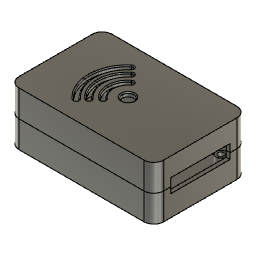
diymore (Autodesk Fusion 360 design; units mm, degrees)
Autodesk Fusion 360 part; units mm, degrees
note: some values were not read from the file. Chosen so that the rebuilt part matches the saved one: which face or edge a step refers to. Set by a fixed rule: which sketch regions a step uses.
sketch "Sketch1" plane through (0, 0, 0) normal (0, 0, 1) x (1, 0, 0) in component "Case"
  line L0 (36.5556, -23.5) -> (-36.5556, -23.5)
  line L1 (-36.5556, -23.5) -> (-36.5556, 23.5)
  line L2 (-36.5556, 23.5) -> (36.5556, 23.5)
  line L3 (36.5556, 23.5) -> (36.5556, -23.5)
  line L4 (36.5556, -23.5) -> (-36.5556, 23.5) construction
  line L5 (-36.5556, -23.5) -> (36.5556, 23.5) construction
  dimension "d4" = 47
  constraint horizontal L0
  constraint perpendicular L0 L1
  constraint parallel L0 L2
  constraint parallel L1 L3
  constraint coincident L4 origin
  constraint coincident L5 origin
  measures "d4" distance of L0.end L1.end
extrude "Extrude1" add sketch "Sketch1" along normal blind 27 makes body 1 in component "Case"
fillet "Fillet1" radius 5 4 edges at (36.5556, -23.5, 13.5) (36.5556, 23.5, 13.5) (-36.5556, -23.5, 13.5) (-36.5556, 23.5, 13.5) on bodies 1 in component "Case"
shell "Shell1" thickness 2 removed faces 0 bodies 1 in component "Case"
ref_plane "WorkPlane1" through (0, 0, 13.5) normal (0, 0, 1) x (1, 0, 0) in component "Case"
sketch "Sketch3" plane through (36.5556, 0, 0) normal (1, 0, 0) x (0, 1, 0) in component "Case"
  line L0 (-18.5, 27) -> (-18.5, 0)
  line L1 (18.5, 0) -> (18.5, 27)
  line L2 (0, 0) -> (0, 7) construction
  line L3 (0, 7) -> (15, 7) construction
  line L4 (0, 7) -> (0, 13.5) construction
  line L5 (0, 7) -> (-15, 7) construction
  line L6 (-13.9847, 14) -> (14, 14) construction
  line L7 (15.0076, 10.5) -> (-14.9924, 10.5)
  line L8 (-14.9924, 10.5) -> (-14.9924, 17.5)
  line L9 (-14.9924, 17.5) -> (15.0076, 17.5)
  line L10 (15.0076, 17.5) -> (15.0076, 10.5)
  line L11 (15.0076, 10.5) -> (-14.9924, 17.5) construction
  line L12 (-14.9924, 10.5) -> (15.0076, 17.5) construction
  line L13 (18.5, 27) -> (-18.5, 27)
  line L14 (-18.5, 0) -> (18.5, 0)
  point P0 (0.0076, 14)
  dimension "d19" = 7
  dimension "d20" = 15
  dimension "d21" = 15
  dimension "d24" = 30
  dimension "d25" = 7
  constraint coincident L2.start origin
  constraint perpendicular L2 L3
  constraint perpendicular L2 L5
  constraint horizontal L6
  constraint horizontal L7
  constraint perpendicular L7 L8
  constraint parallel L7 L9
  constraint parallel L8 L10
  constraint coincident L11 P0
  constraint coincident L12 P0
  constraint midpoint L6 P0
  measures "d19" distance of L2.start L2.end
  measures "d20" distance of L2.end L3.end
  measures "d21" distance of L2.end L5.end
  measures "d24" distance of L8.end L9.end
  measures "d25" distance of L7.end L8.end
extrude "Extrude10" cut sketch "Sketch3" against normal blind 15 contours L7 L8 L9 L10 bodies 1 in component "Case"
sketch "Sketch10" plane through (-36.5556, 0, 0) normal (-1, 0, 0) x (0, -1, 0) in component "Case"
  line L0 (18.5, 0) -> (18.5, 27)
  line L1 (-18.5, 27) -> (-18.5, 0)
  line L2 (14.9924, 17.5) -> (-15.0076, 17.5)
  line L3 (-15.0076, 10.5) -> (14.9924, 10.5)
  line L4 (-5, 17.5) -> (5, 17.5)
  line L5 (5, 17.5) -> (5, 10.5)
  line L6 (5, 10.5) -> (-5, 10.5)
  line L7 (-5, 10.5) -> (-5, 17.5)
  line L8 (-5, 17.5) -> (5, 10.5) construction
  line L9 (5, 17.5) -> (-5, 10.5) construction
  line L10 (-18.5, 0) -> (18.5, 0)
  line L11 (18.5, 27) -> (-18.5, 27)
  point P0 (0, 14)
  dimension "d75" = 10
  constraint horizontal L4
  constraint perpendicular L4 L5
  constraint parallel L4 L6
  constraint parallel L5 L7
  constraint coincident L8 P0
  constraint coincident L9 P0
  measures "d75" distance of L5.end L6.end
extrude "Extrude11" cut sketch "Sketch10" against normal blind 15 contours L2 L3 L4 L5 L6 L7 bodies 1 in component "Case"
split "Split1" by plane through (0, 0, 13.5) normal (0, 0, 1) bodies 1 makes body 2 at (-10.5185, -7.8333, 27) in component "Case"
sketch "Sketch2" plane through (0, 0, 2) normal (0, 0, 1) x (-1, 0, 0) in component "Case"
  circle A0 centre (30, 18) radius 1.5
  circle A1 centre (30, 18) radius 2.5
  circle A2 centre (-29.4798, -17.5013) radius 1.5
  circle A3 centre (-29.4798, -17.5013) radius 2.5
  circle A4 centre (30, -18) radius 1.5
  line L0 (-29.4798, -17.5013) -> (-29.4798, 19.4069) construction
  circle A5 centre (-29.4798, 17.9693) radius 1.5
  arc A6 (-31.5556, 21.5) -> (-34.5556, 18.5) centre (-31.5556, 18.5) ccw
  line L1 (-34.5556, 18.5) -> (-34.5556, -18.5)
  arc A7 (-34.5556, -18.5) -> (-31.5556, -21.5) centre (-31.5556, -18.5) ccw
  line L2 (-31.5556, -21.5) -> (31.5556, -21.5)
  arc A8 (31.5556, -21.5) -> (34.5556, -18.5) centre (31.5556, -18.5) ccw
  line L3 (34.5556, -18.5) -> (34.5556, 18.5)
  arc A9 (34.5556, 18.5) -> (31.5556, 21.5) centre (31.5556, 18.5) ccw
  line L4 (31.5556, 21.5) -> (-31.5556, 21.5)
  dimension "d10" = 3
  dimension "d11" = 1
  dimension "d12" = 3
  dimension "d13" = 1
  dimension "d14" = 3
  dimension "d16" = 3
  constraint coincident A2.centre A3.centre
  constraint vertical L0
  constraint coincident L0 A5.centre
  measures "d10" diameter of A0
  measures "d12" diameter of A2
  measures "d14" diameter of A4
  measures "d16" diameter of A5
extrude "Extrude2" add sketch "Sketch2" along normal blind 6 contours A1 | A3 | A4 | A5 bodies 1 in component "Case"
sketch "Sketch5" plane through (0, 23.5, 0) normal (0, 1, 0) x (-1, 0, 0) in component "Case"
  line L0 (-31.5556, 13.5) -> (-31.5556, 0)
  line L1 (31.5556, 0) -> (31.5556, 13.5)
  line L2 (20.224, 13.5) -> (20.224, 9.5) construction
  line L3 (20.224, 9.5) -> (26.224, 9.5)
  line L4 (26.224, 9.5) -> (26.224, 6.5)
  line L5 (26.224, 6.5) -> (20.224, 6.5)
  line L6 (20.224, 6.5) -> (20.224, 9.5)
  line L7 (31.5556, 13.5) -> (-31.5556, 13.5)
  line L8 (-31.5556, 0) -> (31.5556, 0)
  dimension "d32" = 4
  dimension "d33" = 6
  dimension "d34" = 3
  constraint horizontal L3
  constraint vertical L4
  constraint horizontal L5
  constraint vertical L6
  measures "d32" distance of L2.start L2.end
  measures "d33" distance of L2.end L3.end
  measures "d34" distance of L2.end L5.end
sketch "Sketch7" plane through (0, 0, 13.5) normal (0, 0, 1) x (-1, 0, 0) in component "Case"
  arc A0 (35.0556, 18.5) -> (31.5556, 22) centre (31.5556, 18.5) ccw
  line L0 (-31.5556, 22) -> (31.5556, 22)
  arc A1 (-31.5556, 22) -> (-35.0556, 18.5) centre (-31.5556, 18.5) ccw
  line L1 (-35.0556, 15.4924) -> (-35.0556, 18.5)
  line L2 (-36.0556, 15.4924) -> (-35.0556, 15.4924)
  line L3 (-36.0556, 18.5) -> (-36.0556, 15.4924)
  arc A2 (-31.5556, 23) -> (-36.0556, 18.5) centre (-31.5556, 18.5) ccw
  line L4 (31.5556, 23) -> (-31.5556, 23)
  arc A3 (36.0556, 18.5) -> (31.5556, 23) centre (31.5556, 18.5) ccw
  line L5 (36.0556, 5.5) -> (36.0556, 18.5)
  line L6 (35.0556, 5.5) -> (36.0556, 5.5)
  line L7 (35.0556, 18.5) -> (35.0556, 5.5)
  arc A4 (36.5556, 18.5) -> (31.5556, 23.5) centre (31.5556, 18.5) ccw
  line L8 (31.5556, 23.5) -> (-31.5556, 23.5)
  arc A5 (-31.5556, 23.5) -> (-36.5556, 18.5) centre (-31.5556, 18.5) ccw
  line L9 (-36.5556, 18.5) -> (-36.5556, 14.9924)
  line L10 (-36.5556, 14.9924) -> (-34.5556, 14.9924)
  line L11 (-34.5556, 14.9924) -> (-34.5556, 18.5)
  arc A6 (-31.5556, 21.5) -> (-34.5556, 18.5) centre (-31.5556, 18.5) ccw
  line L12 (-31.5556, 21.5) -> (31.5556, 21.5)
  arc A7 (34.5556, 18.5) -> (31.5556, 21.5) centre (31.5556, 18.5) ccw
  line L13 (34.5556, 18.5) -> (34.5556, 5)
  line L14 (34.5556, 5) -> (36.5556, 5)
  line L15 (36.5556, 5) -> (36.5556, 18.5)
  constraint tangent A0 L0
  constraint tangent A1 L1
  constraint tangent L4 A3
  constraint tangent A3 L5
  constraint tangent L3 A2
  constraint tangent L0 A1
  constraint tangent A2 L4
  constraint tangent A0 L7
sketch "Sketch8" plane through (0, 0, 13.5) normal (0, 0, 1) x (-1, 0, 0) in component "Case"
  arc A0 (-35.0556, -18.5) -> (-31.5556, -22) centre (-31.5556, -18.5) ccw
  line L0 (31.5556, -22) -> (-31.5556, -22)
  arc A1 (31.5556, -22) -> (35.0556, -18.5) centre (31.5556, -18.5) ccw
  line L1 (35.0556, -5.5) -> (35.0556, -18.5)
  line L2 (36.0556, -5.5) -> (35.0556, -5.5)
  line L3 (36.0556, -18.5) -> (36.0556, -5.5)
  arc A2 (31.5556, -23) -> (36.0556, -18.5) centre (31.5556, -18.5) ccw
  line L4 (-31.5556, -23) -> (31.5556, -23)
  arc A3 (-36.0556, -18.5) -> (-31.5556, -23) centre (-31.5556, -18.5) ccw
  line L5 (-36.0556, -15.5076) -> (-36.0556, -18.5)
  line L6 (-35.0556, -15.5076) -> (-36.0556, -15.5076)
  line L7 (-35.0556, -18.5) -> (-35.0556, -15.5076)
  arc A4 (31.5556, -23.5) -> (36.5556, -18.5) centre (31.5556, -18.5) ccw
  line L8 (36.5556, -18.5) -> (36.5556, -5)
  line L9 (36.5556, -5) -> (34.5556, -5)
  line L10 (34.5556, -5) -> (34.5556, -18.5)
  arc A5 (31.5556, -21.5) -> (34.5556, -18.5) centre (31.5556, -18.5) ccw
  line L11 (31.5556, -21.5) -> (-31.5556, -21.5)
  arc A6 (-34.5556, -18.5) -> (-31.5556, -21.5) centre (-31.5556, -18.5) ccw
  line L12 (-34.5556, -18.5) -> (-34.5556, -15.0076)
  line L13 (-34.5556, -15.0076) -> (-36.5556, -15.0076)
  line L14 (-36.5556, -15.0076) -> (-36.5556, -18.5)
  arc A7 (-36.5556, -18.5) -> (-31.5556, -23.5) centre (-31.5556, -18.5) ccw
  line L15 (-31.5556, -23.5) -> (31.5556, -23.5)
  constraint tangent L3 A2
  constraint tangent A3 L5
  constraint tangent A1 L1
  constraint tangent A0 L0
  constraint tangent A0 L7
  constraint tangent L0 A1
  constraint tangent A2 L4
  constraint tangent L4 A3
extrude "Extrude7" add sketch "Sketch8" sketch "Sketch7" along normal blind 2 contours A0 L0 A1 L1 L2 L3 A2 L4 A3 L5 L6 L7 of sketch 2 contours A0 L0 A1 L1 L2 L3 A2 L4 A3 L5 L6 L7 bodies 1 in component "Case"
fillet "Fillet5" radius 0.5 22 edges at (-35.0556, -12, 15.5) (-35.5556, -5.5, 15.5) (-36.0556, -12, 15.5) (-34.7375, -21.682, 15.5) (0, -23, 15.5) (34.7375, -21.682, 15.5) (36.0556, -16.9962, 15.5) (35.5556, -15.4924, 15.5) (35.0556, -16.9962, 15.5) (34.0304, -20.9749, 15.5) (0, -22, 15.5) (-34.0304, -20.9749, 15.5) (35.0556, 17.0038, 15.5) (36.0556, 17.0038, 15.5) (34.7375, 21.682, 15.5) (0, 23, 15.5) (-34.7375, 21.682, 15.5) (-36.0556, 12, 15.5) (-35.0556, 12, 15.5) (-34.0304, 20.9749, 15.5) (0, 22, 15.5) (34.0304, 20.9749, 15.5) on bodies 1 in component "Case"
combine "Combine2" operation cut target body 2 tool bodies 1 keep tools in component "Case"
sketch "Sketch9" plane through (0, 0, 27) normal (0, 0, 1) x (-1, 0, 0) in component "Case"
  circle A0 centre (0, 0) radius 3
  circle A1 centre (0, 0) radius 8
  circle A2 centre (0, 0) radius 10
  circle A3 centre (0, 0) radius 13
  circle A4 centre (0, 0) radius 15
  circle A5 centre (0, 0) radius 17.5
  circle A6 centre (0, 0) radius 19.5
  line L0 (-3, 0.0027) -> (14.6884, 17.6911)
  line L1 (-3, 0.0027) -> (22.0151, 0.0027) construction
  line L2 (-3, 0.0027) -> (15.029, -18.0263)
  line L3 (-3, 0.0027) -> (22.4969, 0.0027) construction
  line L4 (30.5556, 5) -> (24.5556, 5)
  line L5 (24.5556, 5) -> (24.5556, -5)
  line L6 (24.5556, -5) -> (30.5556, -5)
  line L7 (30.5556, -5) -> (30.5556, 5)
  line L8 (-31.0556, -15.0076) -> (-25.0556, -15.0076)
  line L9 (-25.0556, -15.0076) -> (-25.0556, 14.9924)
  line L10 (-25.0556, 14.9924) -> (-31.0556, 14.9924)
  line L11 (-31.0556, 14.9924) -> (-31.0556, -15.0076)
  arc A7 (31.5556, -23.5) -> (36.5556, -18.5) centre (31.5556, -18.5) ccw
  line L12 (36.5556, -18.5) -> (36.5556, 18.5)
  arc A8 (36.5556, 18.5) -> (31.5556, 23.5) centre (31.5556, 18.5) ccw
  line L13 (31.5556, 23.5) -> (-31.5556, 23.5)
  arc A9 (-31.5556, 23.5) -> (-36.5556, 18.5) centre (-31.5556, 18.5) ccw
  line L14 (-36.5556, 18.5) -> (-36.5556, -18.5)
  arc A10 (-36.5556, -18.5) -> (-31.5556, -23.5) centre (-31.5556, -18.5) ccw
  line L15 (-31.5556, -23.5) -> (31.5556, -23.5)
  dimension "d58" = 6
  dimension "d59" = 20
  dimension "d60" = 35
  dimension "d61" = 39
  dimension "d62" = 45
  dimension "d63" = 45
  dimension "d68" = 6
  dimension "d69" = 6
  constraint coincident A0.centre A1.centre
  constraint concentric A0 A2
  constraint concentric A1 A3
  constraint concentric A3 A4
  constraint concentric A0 A6
  constraint horizontal L1
  constraint coincident A0 L0.start
  constraint horizontal L3
  constraint horizontal L4
  constraint vertical L5
  constraint horizontal L6
  constraint vertical L7
  constraint horizontal L8
  constraint vertical L9
  constraint horizontal L10
  constraint vertical L11
  measures "d58" diameter of A0
  measures "d59" diameter of A2
  measures "d60" diameter of A5
  measures "d61" diameter of A6
  measures "d62" angle of L0 L1
  measures "d63" angle of L2 L3
  measures "d68" distance of L4.start L4.end
  measures "d69" distance of L8.start L8.end
extrude "Extrude8" cut sketch "Sketch9" against normal up to surface (13.5 mm away) contours A0 L0 L2 | A0 L0 | A0 L2 | A1 A2 L0 L2 | A3 A4 L0 L2 | A5 A6 L0 L2 picked at (6.5789, 6.5964) picked at (9.4769, 10.7195) picked at (16.306, 9.3515) bodies 2 in component "Case"
fillet "Fillet6" radius 1 12 edges at (-12.2083, 15.2055, 26) (-9.0016, 11.9988, 26) (-5.4118, 8.4091, 26) (-3.9561, 6.9534, 26) (-7.5708, 10.568, 26) (-10.7847, 13.7819, 26) (-3.9526, -6.9553, 26) (-7.5676, -10.5703, 26) (-10.7816, -13.7843, 26) (-12.2052, -15.208, 26) (-8.9984, -12.0012, 26) (-5.4085, -8.4112, 26) on bodies 2 in component "Case"
fillet "Fillet7" radius 0.5 17 edges at (-11.5174, 14.5121, 27) (-17.5, -0.0018, 27) (-11.5143, -14.5145, 27) (-19.5, -0.002, 27) (-9.0363, 11.6585, 27) (-8.0771, 10.6193, 27) (-13, -0.0018, 27) (-8.0741, -10.6217, 27) (-9.0332, -11.661, 27) (-15, -0.0021, 27) (-5.4607, 8.1041, 27) (-4.525, 7.0438, 27) (-8, -0.0017, 27) (-4.5219, -7.0459, 27) (-5.4574, -8.1065, 27) (-10, -0.0022, 27) (2.797, -1.0848, 27) on bodies 2 in component "Case"
component "Case" placed x (1, 0, 0) y (0, 1, 0) z (0, 0, 1) at (0, 0, 0)
named bodies: "Bottom", "Top"
